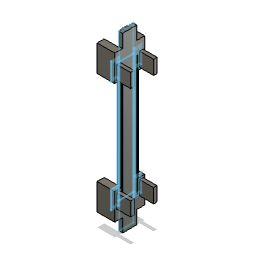
barble_chute_divider_01 (Autodesk Fusion 360 design; units mm, degrees)
Autodesk Fusion 360 part; units mm, degrees
sketch "Sketch1" plane through (0, 0, 0) normal (1, 0, 0) x (0, 0, -1)
  line L0 (-20, 60) -> (-4, 60)
  line L1 (-4, 60) -> (-4, -76)
  line L2 (-4, -76) -> (-20, -76)
  line L3 (-20, -76) -> (-20, 60)
  line L4 (-20, 60) -> (-21, 60)
  line L5 (-21, 60) -> (-21, -76)
  line L6 (-21, -76) -> (-20, -76)
  line L7 (-20, -76) -> (-20, 60)
  line L8 (-4, 60) -> (-3, 60)
  line L9 (-3, 60) -> (-3, -76)
  line L10 (-3, -76) -> (-4, -76)
  line L11 (-4, -76) -> (-4, 60)
  line L12 (-20, 60) -> (-4, 60)
  line L13 (-4, 60) -> (-4, 90)
  line L14 (-4, 90) -> (-20, 90)
  line L15 (-20, 90) -> (-20, 60)
  line L16 (-20, -76) -> (-4, -76)
  line L17 (-4, -76) -> (-4, -106)
  line L18 (-4, -106) -> (-20, -106)
  line L19 (-20, -106) -> (-20, -76)
  line L20 (-20, 60) -> (-21, 60)
  line L21 (-21, 60) -> (-21, 65)
  line L22 (-21, 65) -> (-20, 65)
  line L23 (-20, 65) -> (-20, 60)
  line L24 (-4, 60) -> (-3, 60)
  line L25 (-3, 60) -> (-3, 65)
  line L26 (-3, 65) -> (-4, 65)
  line L27 (-4, 65) -> (-4, 60)
  line L28 (-21, 65) -> (-29, 65)
  line L29 (-29, 65) -> (-29, 45)
  line L30 (-29, 45) -> (-21, 45)
  line L31 (-21, 45) -> (-21, 65)
  line L32 (-3, 65) -> (5, 65)
  line L33 (5, 65) -> (5, 45)
  line L34 (5, 45) -> (-3, 45)
  line L35 (-3, 45) -> (-3, 65)
  line L36 (-21, -76) -> (-20, -76)
  line L37 (-20, -76) -> (-20, -81)
  line L38 (-20, -81) -> (-21, -81)
  line L39 (-21, -81) -> (-21, -76)
  line L40 (-4, -76) -> (-3, -76)
  line L41 (-3, -76) -> (-3, -81)
  line L42 (-3, -81) -> (-4, -81)
  line L43 (-4, -81) -> (-4, -76)
  line L44 (-21, -81) -> (-29, -81)
  line L45 (-29, -81) -> (-29, -61)
  line L46 (-29, -61) -> (-21, -61)
  line L47 (-21, -61) -> (-21, -81)
  line L48 (-3, -81) -> (5, -81)
  line L49 (5, -81) -> (5, -61)
  line L50 (5, -61) -> (-3, -61)
  line L51 (-3, -61) -> (-3, -81)
  line L52 (-21, 45) -> (-22, 45)
  line L53 (-22, 45) -> (-22, -61)
  line L54 (-22, -61) -> (-21, -61)
  line L55 (-21, -61) -> (-21, 45)
  line L56 (-3, -61) -> (-2, -61)
  line L57 (-2, -61) -> (-2, 45)
  line L58 (-2, 45) -> (-3, 45)
  line L59 (-3, 45) -> (-3, -61)
  line L60 (-23, 63) -> (-27, 63)
  line L61 (-27, 63) -> (-27, 47)
  line L62 (-27, 47) -> (-23, 47)
  line L63 (-23, 47) -> (-23, 63)
  line L64 (-1, 63) -> (3, 63)
  line L65 (3, 63) -> (3, 47)
  line L66 (3, 47) -> (-1, 47)
  line L67 (-1, 47) -> (-1, 63)
  line L68 (-23, -79) -> (-27, -79)
  line L69 (-27, -79) -> (-27, -63)
  line L70 (-27, -63) -> (-23, -63)
  line L71 (-23, -63) -> (-23, -79)
  line L72 (-1, -79) -> (3, -79)
  line L73 (3, -79) -> (3, -63)
  line L74 (3, -63) -> (-1, -63)
  line L75 (-1, -63) -> (-1, -79)
  dimension "d1" = 16
  dimension "d2" = 136
  dimension "d3" = 1
  dimension "d4" = 1
  dimension "d5" = 136
  dimension "d6" = 30
  dimension "d7" = 30
  dimension "d8" = 1
  dimension "d9" = 5
  dimension "d10" = 1
  dimension "d11" = 5
  dimension "d12" = 8
  dimension "d13" = 20
  dimension "d14" = 8
  dimension "d15" = 20
  dimension "d16" = 1
  dimension "d17" = 5
  dimension "d18" = 5
  dimension "d19" = 8
  dimension "d20" = 20
  dimension "d21" = 8
  dimension "d22" = 20
  dimension "d23" = 1
  dimension "d24" = 1
  dimension "d25" = 106
  dimension "d26" = -2
  dimension "d27" = 2
  dimension "d28" = 2
  dimension "d29" = -2
  constraint horizontal L0
  constraint vertical L1
  constraint horizontal L2
  constraint vertical L3
  constraint horizontal L4
  constraint vertical L5
  constraint horizontal L6
  constraint vertical L7
  constraint horizontal L8
  constraint vertical L9
  constraint horizontal L10
  constraint vertical L11
  constraint horizontal L12
  constraint vertical L13
  constraint horizontal L14
  constraint vertical L15
  constraint horizontal L16
  constraint vertical L17
  constraint horizontal L18
  constraint vertical L19
  constraint horizontal L20
  constraint vertical L21
  constraint horizontal L22
  constraint vertical L23
  constraint horizontal L24
  constraint vertical L25
  constraint horizontal L26
  constraint vertical L27
  constraint horizontal L28
  constraint vertical L29
  constraint horizontal L30
  constraint vertical L31
  constraint horizontal L32
  constraint vertical L33
  constraint horizontal L34
  constraint vertical L35
  constraint horizontal L36
  constraint vertical L37
  constraint horizontal L38
  constraint vertical L39
  constraint horizontal L40
  constraint vertical L41
  constraint horizontal L42
  constraint vertical L43
  constraint horizontal L44
  constraint vertical L45
  constraint horizontal L46
  constraint vertical L47
  constraint horizontal L48
  constraint vertical L49
  constraint horizontal L50
  constraint vertical L51
  constraint horizontal L52
  constraint vertical L53
  constraint horizontal L54
  constraint vertical L55
  constraint coincident L46 L53.end
  constraint horizontal L56
  constraint vertical L57
  constraint horizontal L58
  constraint vertical L59
  measures "d1" distance of L0.start L0.end
  measures "d2" distance of L0.start L2.end
  measures "d3" distance of L0.start L4.end
  measures "d4" distance of L0.end L8.end
  measures "d5" distance of L0.end L1.end
  measures "d6" distance of L0.start L14.end
  measures "d7" distance of L2.end L18.end
  measures "d8" distance of L0.start L4.end
  measures "d9" distance of L0.start L22.end
  measures "d10" distance of L0.end L8.end
  measures "d11" distance of L0.end L26.end
  measures "d12" distance of L21.end L28.end
  measures "d13" distance of L21.end L30.end
  measures "d14" distance of L25.end L32.end
  measures "d15" distance of L25.end L34.end
  measures "d16" distance of L5.end L2.end
  measures "d17" distance of L5.end L38.end
  measures "d18" distance of L1.end L42.end
  measures "d19" distance of L38.end L44.end
  measures "d20" distance of L38.end L46.end
  measures "d21" distance of L41.end L48.end
  measures "d22" distance of L41.end L50.end
  measures "d23" distance of L30.end L52.end
  measures "d24" distance of L50.end L56.end
  measures "d25" distance of L50.end L34.end
sketch "Sketch2" plane through (0, 0, 0) normal (1, 0, 0) x (0, 0, -1)
extrude "Extrude10" add sketch "Sketch1" along normal blind 4 contours L0 L12 L13 L14 L15 L23 L27 | L0 L1 L2 L3 L7 L11 L12 L16 | L4 L15 L20 L21 L22 L23 L31 | L8 L13 L24 L25 L26 L27 L35 | L6 L19 L36 L37 L38 L39 L47 | L2 L16 L17 L18 L19 L37 L43 | L5 L21 L28 L29 L30 L31 L52 | L10 L17 L40 L41 L42 L43 L51 | L9 L25 L32 L33 L34 L35 L58 | L5 L39 L44 L45 L46 L47 L54 | L5 L30 L46 L52 L53 L54 L55 | L9 L41 L48 L49 L50 L51 L56 | L9 L34 L50 L56 L57 L58 L59 | L60 L61 L62 L63 | L64 L65 L66 L67 | L68 L69 L70 L71 | L72 L73 L74 L75
extrude "Extrude11" add sketch "Sketch1" along normal blind 20 contours L72 L73 L74 L75
extrude "Extrude12" add sketch "Sketch1" along normal blind 20 contours L68 L69 L70 L71
extrude "Extrude13" add sketch "Sketch1" against normal blind 16 contours L9 L41 L48 L49 L50 L51 L56
extrude "Extrude14" add sketch "Sketch1" against normal blind 16 contours L5 L39 L44 L45 L46 L47 L54
extrude "Extrude15" add sketch "Sketch1" along normal blind 20 contours L64 L65 L66 L67
extrude "Extrude16" add sketch "Sketch1" along normal blind 20 contours L60 L61 L62 L63
extrude "Extrude17" add sketch "Sketch1" against normal blind 16 contours L9 L25 L32 L33 L34 L35 L58
extrude "Extrude18" add sketch "Sketch1" against normal blind 16 contours L5 L21 L28 L29 L30 L31 L52
extrude "Extrude19" add 2 faces at (-4, -81, -2.3333) (-4, -81, 26.3333) along direction (0, -1, 0) blind 10
extrude "Extrude20" add 2 faces at (-4, 65, -2.3333) (-4, 65, 26.3333) along direction (0, 1, 0) blind 10
extrude "Extrude21" cut 1 faces at (9.3333, 63, 24.3333) along direction (0, -1, 0) blind 0.1
extrude "Extrude22" cut 1 faces at (9.3333, 57.6, 27) along direction (0, 0, -1) blind 0.1
extrude "Extrude23" cut 1 faces at (14.6667, 63, -0.3333) along direction (0, -1, 0) blind 0.1
extrude "Extrude24" cut 1 faces at (9.3333, 52.3, 1) along direction (0, 0, -1) blind 0.1
extrude "Extrude25" cut 1 faces at (14.6667, -63, -1.6667) along direction (0, -1, 0) blind 0.1
extrude "Extrude26" cut 1 faces at (9.3333, -63, 25.6667) along direction (0, -1, 0) blind 0.1
extrude "Extrude1" [rolled back] along distance -4 taper angle 0
extrude "Extrude2" [rolled back] along distance -4 taper angle 0
extrude "Extrude3" [rolled back] along distance 16 taper angle 0
extrude "Extrude4" [rolled back] along distance 16 taper angle 0
extrude "Extrude5" [rolled back] along distance 16 taper angle 0
extrude "Extrude6" [rolled back] along distance 16 taper angle 0
extrude "Extrude7" [rolled back] along distance -20 taper angle 0
extrude "Extrude8" [rolled back] along distance -20 taper angle 0
extrude "Extrude9" [rolled back] along distance -20 taper angle 0
equation "d25 = 136 mm - 30 mm"
